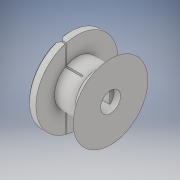
# Autodesk Inventor part: PullingWheel
Saved by Autodesk Inventor 2019 (Build 230136000, 136)
## iProperties
Created: 2018-08-14
Part Number: PullingWheel
Material: Generisch
Document SubType Name: Modeling
Designer: janbe
Density: 1 g/cm^3
Appearance: Vorgabe
Author: janbe
Autodesk Inventor part; units mm, degrees
ref_plane "YZ Plane" through (0, 0, 0) normal (1, 0, 0) x (0, 1, 0)
ref_plane "XZ Plane" through (0, 0, 0) normal (0, 1, 0) x (-1, 0, 0)
ref_plane "XY Plane" through (0, 0, 0) normal (0, 0, 1) x (1, 0, 0)
sketch "Skizze1" plane through (0, 0, 0) normal (0, 0, 1) x (1, 0, 0)
  line L0 (0, 0) -> (11, 0)
  line L1 (11, 0) -> (11, -6)
  line L2 (11, -6) -> (0, -6)
  line L3 (0, -6) -> (0, 0)
  line L4 (0, -6) -> (2, -6)
  line L5 (2, -6) -> (2, -11)
  line L6 (2, -11) -> (0, -11)
  line L7 (0, -11) -> (0, -6)
  line L8 (11, -6) -> (8.5, -6)
  line L9 (7.5, -6) -> (11, -10)
  line L10 (11, -10) -> (11, -6)
  dimension "d0" = 11
  dimension "d1" = 6
  dimension "d2" = 2
  dimension "d3" = 5
  dimension "d5" = 5.5
  dimension "d6" = 4
  constraints: 22 end point, 4 parallel, 3 horizontal, 2 perpendicular, 1 point on line, 1 vertical
  measures "d0" distance of L1.end L2.end
  measures "d1" distance of L0.end L1.end
  measures "d2" distance of L5.end L6.end
  measures "d3" distance between parallel lines of L2 L6
  measures "d5" distance from line of L9.start L5
  measures "d6" distance of L9.end L1.end
revolve "Umdrehung1" add sketch "Skizze1" angle 360 about axis through (0, 0, 0) along (1, 0, 0)
sketch "Skizze3" plane through (11, 0, 0) normal (1, 0, 0) x (0, 0, -1)
  circle A0 centre (0, 0) radius 10 projected
  circle A1 centre (0, 0) radius 11 projected
  circle A2 centre (0.009, 0) radius 2.675
  line L0 (-2.2058, 1.5) -> (2.2239, 1.5)
  line L1 (-2.2058, -1.5) -> (2.2239, -1.5)
  point P0 (17.2536, -1.634)
  dimension "d8" = 5.35
  dimension "d9" = 1.5
  dimension "d10" = 1.5
  constraints: 4 end point, 4 point on circle, 2 coincident, 1 centre point, 1 horizontal, 1 parallel
  measures "d8" diameter of A2
  measures "d9" distance from line of point (0, 0) L0
  measures "d10" distance from line of point (0, 0) L1
extrude "Extrusion1" cut sketch "Skizze3" against normal blind 8.5 contours A2 L1 L0
extrude "Extrusion2" cut sketch "Skizze3" against normal blind 1.7 contours L0 A2 | A2 L1
sketch "Skizze4" plane through (0, 0, 0) normal (-1, 0, 0) x (0, 0, 1)
  circle A0 centre (0, 0) radius 11 projected
  circle A1 centre (0, 0) radius 6 projected
  arc A2 (2.2058, -1.5) -> (2.2058, 1.5) centre (-0.009, 0) ccw projected
  arc A3 (-2.2239, -1.5) -> (2.2058, -1.5) centre (-0.009, 0) ccw projected
  arc A4 (-2.2239, 1.5) -> (-2.2239, -1.5) centre (-0.009, 0) ccw projected
  line L0 (2.2058, 1.5) -> (-2.2239, 1.5) projected
  line L1 (-2.2239, -1.5) -> (2.2058, -1.5) projected
  arc A5 (2.2058, 1.5) -> (-2.2239, 1.5) centre (-0.009, 0) ccw projected
  line L2 (-10.6271, -3.15) -> (10.6271, -3.15)
  line L3 (10.6271, -3.15) -> (10.6271, -2.84)
  line L4 (10.6271, -2.84) -> (-10.6271, -2.84)
  line L5 (-10.6271, -2.84) -> (-10.6271, -3.15)
  circle A6 centre (0, 0) radius 11 projected
  dimension "d15" = 0.31
  dimension "d16" = 2.84
  constraints: 8 end point, 2 parallel, 2 point on circle, 1 horizontal, 1 perpendicular
  measures "d15" distance of L4.end L2.start
  measures "d16" distance from line of point (0, 0) L4
extrude "Extrusion3" cut sketch "Skizze4" against normal blind 6.5 contours L4 A1 L2 A0 | A0 L2 L5 | L3 L2 A0 | A0 L2 A1 L4 | L4 A1 L2
chamfer "Fase1" distance 1 angle 45 2 edges at (0, -2.84, 0) (0, -3.15, 0)
chamfer "Fase2" distance 0.3 angle 45 2 edges at (0, -11, 0) (0, 11, 0)
sketch "Skizze5" plane through (0, 0, 0) normal (0, 1, 0) x (-1, 0, 0)
  circle A0 centre (-4.5, 0) radius 1.8
  line L0 (0, 10.7) -> (0, -10.7) projected
  point P0 (0, 0)
  point P1 (0, -10.5406)
  point P2 (0, 10.5406)
  dimension "d25" = 3.6
  dimension "d26" = 4.5
  constraints: 1 centre point
  measures "d25" diameter of A0
  measures "d26" distance from line of A0.centre L0
extrude "Extrusion4" [suppressed]
